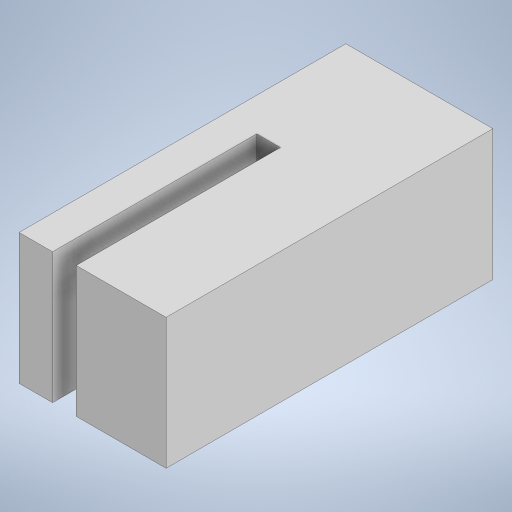
# Autodesk Inventor part: PCB_Holder
Saved by Autodesk Inventor 2023 (Build 270158000, 158)
## iProperties
Created: 2022-12-11
Part Number: PCB_Holder
Material: Generic
Document SubType Name: Modeling
Designer: spfow
Density: 1 g/cm^3
Appearance: Default
Author: spfow
Autodesk Inventor part; units mm, degrees
ref_plane "YZ Plane" through (0, 0, 0) normal (1, 0, 0) x (0, 1, 0)
ref_plane "XZ Plane" through (0, 0, 0) normal (0, 1, 0) x (-1, 0, 0)
ref_plane "XY Plane" through (0, 0, 0) normal (0, 0, 1) x (1, 0, 0)
sketch "Sketch1" plane through (0, 0, 0) normal (0, 1, 0) x (-1, 0, 0)
  line L0 (0, 0) -> (11.43, 0)
  line L1 (11.43, 0) -> (11.43, -25.4)
  line L2 (11.43, -25.4) -> (0, -25.4)
  line L3 (0, -25.4) -> (0, 0)
  dimension "d0" = 11.43
  dimension "d1" = 25.4
  constraints: 8 end point, 2 parallel, 1 horizontal, 1 perpendicular
  measures "d0" distance of L1.end L2.end
  measures "d1" distance of L0.end L1.end
extrude "Extrusion1" add sketch "Sketch1" along normal blind 10.16
sketch "Sketch2" plane through (0, 10.16, 0) normal (0, 1, 0) x (1, 0, 0)
  line L0 (0, 0) -> (0, 25.4) projected
  line L1 (0, 0) -> (-6.985, 0)
  line L2 (-6.985, 0) -> (-6.985, 4.6296)
  line L3 (-6.985, 4.6296) -> (0, 4.6296)
  line L4 (0, 4.6296) -> (0, 0)
  line L5 (-6.985, 0) -> (-8.8265, 0)
  line L6 (-8.8265, 0) -> (-8.8265, 15.875)
  line L7 (-8.8265, 15.875) -> (-6.985, 15.875)
  line L8 (-6.985, 15.875) -> (-6.985, 0)
  dimension "d4" = 6.985
  dimension "d5" = 1.8415
  dimension "d6" = 15.875
  constraints: 16 end point, 4 parallel, 2 horizontal, 2 perpendicular
  measures "d4" distance of L2.end L3.end
  measures "d5" distance of L6.end L7.end
  measures "d6" distance of L5.end L6.end
extrude "Extrusion2" cut sketch "Sketch2" against normal blind 12.7 contours L5 L6 L7 L8 L2
body "Solid1"
